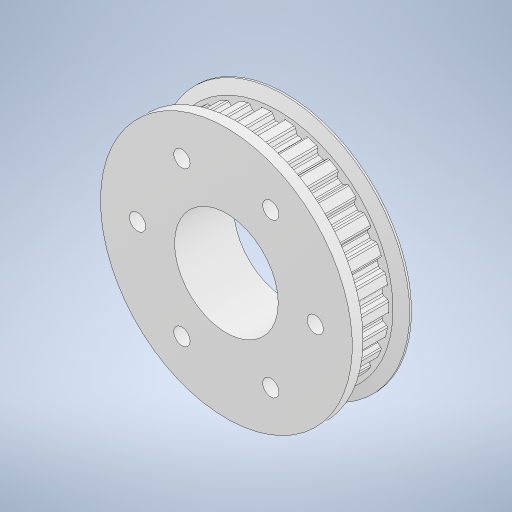
# Autodesk Inventor part: XL Belt Generator
Saved by Autodesk Inventor 2023.4 (Build 274418000, 418)
## iProperties
RuleStatus: InUse
Created: 2022-06-22
Part Number: XL Belt Generator
Material: UHMW, White
Document SubType Name: Modeling
Designer: Nathan Cai
Density: 0.94 g/cm^3
Appearance: Smooth - White
Mass: 3.49489 g
Surface Area: 67.8029 cm^2
Volume: 3.75794 cm^3
Author: Nathan Cai
Autodesk Inventor part; units mm, degrees
ref_plane "YZ Plane" through (0, 0, 0) normal (1, 0, 0) x (0, 1, 0)
ref_plane "XZ Plane" through (0, 0, 0) normal (0, 1, 0) x (-1, 0, 0)
ref_plane "XY Plane" through (0, 0, 0) normal (0, 0, 1) x (1, 0, 0)
sketch "Sketch2" plane through (0, 0, 0) normal (0, 0, 1) x (1, 0, 0)
  circle A0 centre (0, 0) radius 24.2552 construction
  circle A1 centre (0, 0) radius 23.7402
  dimension "Pd" = 48.5104
  dimension "OD" = 47.4804
  constraints: 2 centre point, 2 coincident
  measures "Pd" diameter of A0
  measures "OD" diameter of A1
extrude "Extrusion3" add sketch "Sketch2" along normal blind 7.62
sketch "Sketch3" plane through (0, 0, 7.62) normal (0, 0, 1) x (1, 0, 0)
  line L0 (0, 0) -> (0, 23.7402) construction
  circle A0 centre (0, 0) radius 23.7402 projected
  line L1 (0, 0) -> (4.9359, 23.2214) construction
  circle A1 centre (0, 0) radius 22.4702
  line L2 (0.8085, 22.6849) -> (1.1752, 23.4713)
  line L3 (1.2844, 23.7054) -> (0, 0) construction
  arc A2 (1.5443, 23.6899) -> (1.1752, 23.4713) centre (1.5196, 23.3107) ccw
  arc A3 (0.4564, 22.4656) -> (0.8085, 22.6849) centre (0.4641, 22.8455) ccw
  circle A4 centre (0, 0) radius 23.7402 projected
  line L4 (-0.8085, 22.6849) -> (-1.1752, 23.4713)
  arc A5 (-1.1752, 23.4713) -> (-1.5443, 23.6899) centre (-1.5196, 23.3107) ccw
  arc A6 (-0.8085, 22.6849) -> (-0.4564, 22.4656) centre (-0.4641, 22.8455) ccw
  point P0 (2.2035, 22.3619)
  point P1 (1.5443, 23.6899)
  point P2 (-1.5443, 23.6899)
  point P3 (-0.4564, 22.4656)
  dimension "d29" = 12
  dimension "d30" = 44.9404
  dimension "d31" = 25
  dimension "d33" = 3.101
  dimension "d34" = 0.76
  dimension "d35" = 0.76
  constraints: 14 point on circle, 10 end point, 6 symmetric about line, 5 centre point, 4 tangent, 1 coincident, 1 point on line, 1 vertical, 2 other
  measures "d29" angle of L0 L1
  measures "d30" diameter of A1
  measures "d31" angle of L0 L2
  measures "d33" angle of L0 L3
  measures "d34" diameter of A2
  measures "d35" diameter of A3
extrude "Extrusion4" cut sketch "Sketch3" against normal through all contours A2 L2 A3 A1 A6 L4 A5 A0 picked at (-0.0507, 23.313)
pattern_circular "Circular Pattern2" count 30 over 360 about axis through (0, 0, 0) along (0, 0, 1) of "Extrusion4"
ref_plane "Work Plane1" through (0, 0, 3.81) normal (0, 0, 1) x (1, 0, 0)
sketch "Sketch4" plane through (0, 0, 7.62) normal (0, 0, 1) x (1, 0, 0)
  circle A0 centre (0, 0) radius 26.9875
  dimension "d42" = 53.975
  constraints: 1 centre point, 1 coincident
  measures "d42" diameter of A0
extrude "Extrusion5" add sketch "Sketch4" along normal blind 1.5875
chamfer "Chamfer1" distance 1.1906 distance2 2.3813 1 edges at (-26.9875, 0, 7.62) measured on face at (-26.9875, 0, 8.12)
mirror "Mirror1" about plane through (0, 0, 3.81) normal (0, 0, 1) of "Extrusion5", "Chamfer1"
thicken "Thicken1" operation add thickness 1.905 both sides no extend neighbours no toward (0, 0, 1) faces at (3.19, 8.4113, 9.2075)
sketch "Sketch5" plane through (0, 0, -1.5875) normal (0, 0, -1) x (-1, 0, 0)
  circle A0 centre (0, 0) radius 11.1125
  circle A1 centre (0, 0) radius 19.05 construction
  line L0 (0, 0) -> (19.05, 0) construction
  circle A2 centre (19.05, 0) radius 1.7526
  circle A3 centre (9.525, 16.4978) radius 1.7526
  circle A4 centre (-9.525, 16.4978) radius 1.7526
  circle A5 centre (-19.05, 0) radius 1.7526
  circle A6 centre (-9.525, -16.4978) radius 1.7526
  circle A7 centre (9.525, -16.4978) radius 1.7526
  dimension "d51" = 38.1
  dimension "d50" = 22.225
  dimension "d52" = 3.5052
  dimension "d55" = 360
  constraints: 7 centre point, 3 coincident, 2 end point, 1 horizontal, 1 horizontal alignment, 15 other
  measures "d50" diameter of A0
  measures "d52" diameter of A2
extrude "Extrusion6" cut sketch "Sketch5" against normal through all
equation "\"pitch\" = 5.08"
equation "\"width\" = 7.62"
equation "\"T_angle\" = 50deg"
equation "\"T_ht\" = 1.27"
equation "\"r1\" = 0.38"
equation "\"r2\" = 0.38"
equation "\"T_hs\" = 2.3"
equation "\"T_s\" = 2.57"
body "Solid3"
